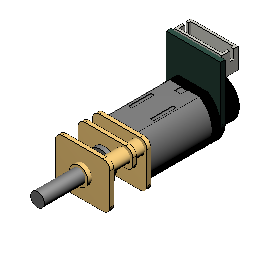
lf (Autodesk Fusion 360 archive; units mm, degrees)
design "N20-enc"
Autodesk Fusion 360 part; units mm, degrees
note: some values were not read from the file. Chosen so that the rebuilt part matches the saved one: a direction. Set by a fixed rule: which sketch regions a step uses.
sketch "Sketch1" plane through (0, 0, 0) normal (0, 1, 0) x (1, 0, 0)
  line L0 (-3.25, -5) -> (3.25, -5)
  arc A0 (3.25, -5) -> (3.25, 5) centre (0.0795, 0) ccw
  line L1 (3.25, 5) -> (-3.25, 5)
  arc A1 (-3.25, 5) -> (-3.25, -5) centre (-0.0795, 0) ccw
  line L2 (0, 0) -> (0, -6) construction
  line L3 (0, 0) -> (10, 0) construction
  dimension "d1" = 10
  dimension "d2" = 12
  dimension "d3" = 6.5
  constraint horizontal L0
  constraint horizontal L1
  constraint coincident L2.start L3.start
  constraint vertical L2
  constraint perpendicular L2 L3
  constraint symmetric L0 L1 L3
  constraint symmetric A0 A1 L2
  constraint equal L0 L1
  measures "d1" distance of L0 L1
  measures "d3" distance of L0.start L0.end
extrude "Extrude1" add sketch "Sketch1" along normal blind 13.5 makes body 1
extrude "Extrude2" add 1 faces at (1.0833, 13.5, -1.6667) along direction (0, 1, 0) blind 2 separate body on bodies 1 makes body 2
sketch "Sketch3" plane through (0, 0, 0) normal (0, -1, 0) x (1, 0, 0)
  arc A0 (-3.25, 5) -> (-3.25, -5) centre (-0.0795, 0) ccw
  line L0 (-3.25, -5) -> (3.25, -5)
  arc A1 (3.25, -5) -> (3.25, 5) centre (0.0795, 0) ccw
  line L1 (3.25, 5) -> (-3.25, 5)
  line L2 (-4.5, 5) -> (4.5, 5)
  line L3 (6, 3.5) -> (6, -3.5)
  line L4 (4.5, -5) -> (-4.5, -5)
  line L5 (-6, -3.5) -> (-6, 3.5)
  line L6 (0, 0) -> (0, 5) construction
  line L7 (0, 0) -> (6, 0) construction
  arc A2 (-4.5, 5) -> (-6, 3.5) centre (-4.5, 3.5) ccw
  arc A3 (6, 3.5) -> (4.5, 5) centre (4.5, 3.5) ccw
  arc A4 (4.5, -5) -> (6, -3.5) centre (4.5, -3.5) ccw
  arc A5 (-6, -3.5) -> (-4.5, -5) centre (-4.5, -3.5) ccw
  point P0 (-6, 5)
  point P1 (6, 5)
  point P2 (-6, -5)
  dimension "d8" = 12
  dimension "d9" = 10
  dimension "d10" = 1.5
  constraint horizontal L2
  constraint vertical L3
  constraint horizontal L4
  constraint vertical L5
  constraint vertical L6
  constraint coincident L6.start L7.start
  constraint perpendicular L3 L7
  constraint coincident L2 L6.end
  constraint coincident P0 L2
  constraint coincident P0 L5
  constraint tangent L2 A2
  constraint tangent L5 A2
  constraint coincident L3 L7.end
  constraint coincident P1 L2
  constraint coincident P1 L3
  constraint tangent L2 A3
  constraint tangent L3 A3
  constraint equal A2 A3
  constraint tangent L3 A4
  constraint tangent L4 A4
  constraint equal A2 A4
  constraint coincident P2 L4
  constraint coincident P2 L5
  constraint tangent L4 A5
  constraint tangent L5 A5
  constraint equal A2 A5
  constraint midpoint L2 L6.end
  constraint midpoint L3 L7.end
  measures "d8" distance of P0 P1
  measures "d9" distance of P0 P2
  measures "d10" radius of A2
extrude "Extrude3" add sketch "Sketch3" along normal blind 0.8 separate body makes body 3
sketch "Sketch4" plane through (0, 15.5, 0) normal (0, 1, 0) x (-1, 0, 0)
  arc A0 (3.25, -5) -> (3.25, 5) centre (0.0795, 0) ccw
  line L0 (3.25, 5) -> (-3.25, 5)
  arc A1 (-3.25, 5) -> (-3.25, -5) centre (-0.0795, 0) ccw
  line L1 (-6, 12) -> (-6, -1.5)
  line L2 (-6, 3.5) -> (-6, -3.5) construction
  line L3 (6, -3.5) -> (6, 3.5) construction
  line L4 (6, 12) -> (6, -1.5)
  line L5 (-6, 12) -> (6, 12)
  line L6 (-3.25, -5) -> (3.25, -5) construction
  line L7 (-4.25, -5) -> (4.25, -5)
  line L8 (-6, -1.5) -> (-4.25, -5)
  line L9 (4.25, -5) -> (6, -1.5)
  line L10 (0, 0) -> (0, 14.3086) construction
  circle A2 centre (0, 0) radius 1
  dimension "d13" = 17
  dimension "d14" = 8.5
  dimension "d15" = 13.5
  dimension "d18" = 2
  constraint vertical L1
  constraint collinear L1 L2
  constraint vertical L4
  constraint collinear L3 L4
  constraint horizontal L5
  constraint horizontal L7
  constraint collinear L6 L7
  constraint coincident L10.start A2.centre
  constraint vertical L10
  constraint symmetric L8 L9 L10
  measures "d13" distance of L5 L7
  measures "d14" distance of L7.start L7.end
  measures "d15" distance of L1.start L1.end
  measures "d18" diameter of A2
extrude "Extrude4" add sketch "Sketch4" along normal blind 1 separate body contours A0 L0 A1 L7 | A0 L0 A1 L1 L4 L5 makes body 4
sketch "Sketch5" plane through (0, 0, 0) normal (1, 0, 0) x (0, 1, 0)
  line L0 (24.2202, 0) -> (0, 0) construction
  line L1 (15, 0.5) -> (17.5, 0.5)
  line L2 (17.5, 0.5) -> (17.5, 4.6)
  line L3 (17.5, 4.6) -> (21, 4.6)
  line L4 (21, 4.6) -> (21, 2.6)
  line L5 (21, 2.6) -> (20.7, 1.5)
  line L6 (20.7, 1.5) -> (20.7, 0)
  line L7 (15, 0) -> (15, 0.5)
  line L8 (15, 0) -> (20.7, 0)
  dimension "d19" = 0.5
  dimension "d20" = 4.6
  dimension "d21" = 3.5
  dimension "d22" = 2
  dimension "d23" = 1.5
  dimension "d24" = 0.3
  dimension "d25" = 21
  dimension "d26" = 15
  constraint coincident L0.end origin
  constraint horizontal L0
  constraint parallel L0 L1
  constraint perpendicular L1 L2
  constraint perpendicular L2 L3
  constraint perpendicular L3 L4
  constraint coincident L0 L6.end
  constraint perpendicular L0 L6
  constraint coincident L0 L7.start
  constraint perpendicular L1 L7
  measures "d19" distance of L0 L1
  measures "d20" distance of L0 L3
  measures "d21" distance of L2.end L3.end
  measures "d22" distance of L3.end L4.end
  measures "d23" distance of L5.end L6.end
  measures "d24" distance of L4 L6
  measures "d25" distance of L0.end L4
  measures "d26" distance of L0.end L7
revolve "Revolve1" add sketch "Sketch5" angle 360 about axis through (0, 24.2202, 0) along (0, -1, 0) separate body makes body 5
sketch "Sketch6" plane through (0, 0, 0) normal (0, 1, 0) x (1, 0, 0)
  arc A0 (-4.5, 5) -> (-6, 3.5) centre (-4.5, 3.5) ccw
  line L0 (-6, 3.5) -> (-6, -3.5)
  arc A1 (-6, -3.5) -> (-4.5, -5) centre (-4.5, -3.5) ccw
  line L1 (-4.5, -5) -> (4.5, -5)
  arc A2 (4.5, -5) -> (6, -3.5) centre (4.5, -3.5) ccw
  line L2 (6, -3.5) -> (6, 3.5)
  arc A3 (6, 3.5) -> (4.5, 5) centre (4.5, 3.5) ccw
  line L3 (4.5, 5) -> (-4.5, 5)
  circle A4 centre (-4, 3) radius 1.5
  circle A5 centre (4, -3) radius 1.5
  arc A6 (-6, -3.5) -> (-4.5, -5) centre (-4.5, -3.5) ccw
  line L4 (-4.5, -5) -> (4.5, -5)
  arc A7 (4.5, -5) -> (6, -3.5) centre (4.5, -3.5) ccw
  line L5 (6, -3.5) -> (6, 3.5)
  arc A8 (6, 3.5) -> (4.5, 5) centre (4.5, 3.5) ccw
  line L6 (4.5, 5) -> (-4.5, 5)
  arc A9 (-4.5, 5) -> (-6, 3.5) centre (-4.5, 3.5) ccw
  line L7 (-6, 3.5) -> (-6, -3.5)
  dimension "d29" = 3
  dimension "d32" = 0.5
  dimension "d33" = 0.5
  dimension "d38" = 0.5
  dimension "d39" = 0.5
  constraint equal A4 A5
  measures "d29" diameter of A5
  measures "d32" distance of L2 A5
  measures "d33" distance of L0 A4
  measures "d38" distance of L3 A4
  measures "d39" distance of L1 A5
extrude "Extrude5" add sketch "Sketch6" against normal blind 8.5 from surface at -0.5 contours A4 | A5 bodies 3
sketch "Sketch8" plane through (0, -0.8, 0) normal (0, -1, 0) x (-1, 0, 0)
  line L0 (6, 3.5) -> (6, -3.5)
  arc A0 (6, 3.5) -> (4.5, 5) centre (4.5, 3.5) ccw
  arc A1 (-6, -3.5) -> (-4.5, -5) centre (-4.5, -3.5) ccw
  line L1 (4.5, -5) -> (-4.5, -5)
  arc A2 (4.5, -5) -> (6, -3.5) centre (4.5, -3.5) ccw
  line L2 (-1.0827, 4.0905) -> (-1.4214, 0.3651)
  line L3 (-2.2932, -0.5367) -> (-5.124, -0.8905)
  line L4 (4.5, 5) -> (-0.0868, 5)
  line L5 (-6, -3.5) -> (-6, -1.8828)
  arc A3 (-5.124, -0.8905) -> (-6, -1.8828) centre (-5, -1.8828) ccw
  arc A4 (-2.2932, -0.5367) -> (-1.4214, 0.3651) centre (-2.4172, 0.4556) ccw
  arc A5 (-0.0868, 5) -> (-1.0827, 4.0905) centre (-0.0868, 4) ccw
  point P0 (-1, 5)
  point P1 (-6, -1)
  dimension "d49" = 7
  dimension "d50" = 4
  dimension "d51" = 1
  constraint coincident A0.end L4.start
  constraint coincident A1.start L5.start
  constraint tangent A1 L5
  constraint coincident P1 L3
  constraint coincident P1 L5
  constraint tangent L3 A3
  constraint tangent L5 A3
  constraint tangent L2 A4
  constraint tangent L3 A4
  constraint equal A3 A4
  constraint coincident P0 L2
  constraint coincident P0 L4
  constraint tangent L2 A5
  constraint tangent L4 A5
  constraint equal A3 A5
  measures "d49" distance of L0 P0
  measures "d50" distance of L1 P1
  measures "d51" radius of A3
extrude "Extrude6" add sketch "Sketch8" along normal blind 0.8 from surface at 2.4 bodies 3
extrude "Extrude7" add sketch "Sketch3" against normal blind 0.8 from surface at 9 bodies 3
sketch "Sketch9" plane through (0, -9, 0) normal (0, -1, 0) x (1, 0, 0)
  line L0 (4.5, 5) -> (-4.5, 5)
  arc A0 (-4.5, 5) -> (-6, 3.5) centre (-4.5, 3.5) ccw
  line L1 (-6, 3.5) -> (-6, -3.5)
  arc A1 (-6, -3.5) -> (-4.5, -5) centre (-4.5, -3.5) ccw
  line L2 (-4.5, -5) -> (4.5, -5)
  arc A2 (4.5, -5) -> (6, -3.5) centre (4.5, -3.5) ccw
  line L3 (6, -3.5) -> (6, 3.5)
  arc A3 (6, 3.5) -> (4.5, 5) centre (4.5, 3.5) ccw
  circle A4 centre (0, 0) radius 2
  dimension "d55" = 4
  constraint coincident A4.centre origin
  measures "d55" diameter of A4
extrude "Extrude8" add sketch "Sketch9" along normal blind 0.9 contours A4 bodies 3
sketch "Sketch10" plane through (0, 0, 0) normal (1, 0, 0) x (0, 1, 0)
  line L0 (-19, 1.5) -> (-8.2, 1.5)
  line L1 (-19, 0) -> (-19, 1.5)
  line L2 (-8.2, 1.5) -> (-8.2, 2)
  line L3 (-8.2, 2) -> (-5.2, 2)
  line L4 (0, 0) -> (-19, 0) construction
  line L5 (-4.2, 2.75) -> (-5.2, 2.75)
  line L6 (-4.2, 0.5) -> (-3.2, 0.5)
  line L7 (-3.2, 0.5) -> (-3.2, 0)
  line L8 (-5.2, 2.75) -> (-5.2, 2)
  line L9 (-3.2, -3.5) -> (-3.2, 3.5) construction
  line L10 (-4, 3.5) -> (-4, -3.5) construction
  line L11 (-8.2, -3.5) -> (-8.2, 3.5) construction
  line L12 (-9, -3.5) -> (-9, 3.5) construction
  line L13 (-4.2, 0.5) -> (-4.2, 2.75)
  line L14 (-19, 0) -> (-3.2, 0)
  dimension "d62" = 3
  dimension "d64" = 10
  dimension "d65" = 1.5
  dimension "d66" = 2
  dimension "d67" = 2.75
  dimension "d68" = 0.5
  dimension "d69" = 0.2
  constraint horizontal L0
  constraint vertical L1
  constraint perpendicular L0 L2
  constraint coincident L4.start origin
  constraint horizontal L5
  constraint vertical L8
  constraint horizontal L6
  constraint vertical L7
  constraint collinear L7 L9
  constraint collinear L2 L11
  measures "d62" distance of L2 L8
  measures "d64" distance of L1 L12
  measures "d65" distance of L0 L4
  measures "d66" distance of L3 L14
  measures "d67" distance of L4 L5
  measures "d68" distance of L6 L14
  measures "d69" distance of L10 L13
revolve "Revolve2" add sketch "Sketch10" angle 360 about axis through (0, 0, 0) along (0, -1, 0) separate body makes body 6
sketch "Sketch11" plane through (0, 16.5, 0) normal (0, 1, 0) x (-1, 0, 0)
  circle A0 centre (0, 0) radius 1
  line L0 (-6, 12) -> (-6, 0)
  arc A1 (-6, 0) -> (-3.25, -5) centre (-0.0795, 0) ccw
  line L1 (-3.25, -5) -> (3.25, -5)
  arc A2 (3.25, -5) -> (6, 0) centre (0.0795, 0) ccw
  line L2 (6, 0) -> (6, 12)
  line L3 (6, 12) -> (-6, 12)
  line L4 (-5.25, 12.4) -> (5.25, 12.4)
  line L5 (5.25, 12.4) -> (5.25, 7.9)
  line L6 (5.25, 7.9) -> (-5.25, 7.9)
  line L7 (-5.25, 7.9) -> (-5.25, 12.4)
  line L8 (0, 0) -> (0, 18.1441) construction
  dimension "d71" = 4.5
  dimension "d72" = 10.5
  dimension "d73" = 0.4
  constraint horizontal L4
  constraint vertical L5
  constraint horizontal L6
  constraint vertical L7
  constraint coincident A0.centre L8.start
  constraint vertical L8
  constraint symmetric L5 L7 L8
  measures "d71" distance of L4.end L5.end
  measures "d72" distance of L4.start L4.end
  measures "d73" distance of L3 L4
extrude "Extrude9" add sketch "Sketch11" along normal blind 3.6 separate body contours L3 L4 L5 L7 | L3 L5 L6 L7 makes body 7
sketch "Sketch12" plane through (0, 0, 12.4) normal (0, 0, 1) x (-1, 0, 0)
  line L0 (5.25, -16.5) -> (-5.25, -16.5)
  line L1 (-5.25, -16.5) -> (-5.25, -20.1)
  line L2 (-5.25, -20.1) -> (5.25, -20.1)
  line L3 (5.25, -20.1) -> (5.25, -16.5)
  line L4 (4.75, -19.6) -> (4.75, -17)
  line L5 (4.75, -17) -> (-4.75, -17)
  line L6 (-4.75, -17) -> (-4.75, -19.6)
  line L7 (-4.75, -19.6) -> (4.75, -19.6)
  dimension "d76" = -0.5
extrude "Extrude10" cut sketch "Sketch12" against normal blind 3.3 contours L4 L5 L6 L7 bodies 7
sketch "Sketch13" plane through (5.25, 0, 0) normal (1, 0, 0) x (0, 1, 0)
  line L0 (16.5, 7.9) -> (20.1, 7.9)
  line L1 (20.1, 7.9) -> (20.1, 12.4)
  line L2 (20.1, 12.4) -> (16.5, 12.4)
  line L3 (16.5, 12.4) -> (16.5, 7.9)
  line L4 (18.25, 12.4) -> (19.1, 12.4)
  line L5 (19.1, 12.4) -> (19.1, 10.4)
  line L6 (19.1, 10.4) -> (18.25, 10.4)
  line L7 (18.25, 10.4) -> (18.25, 12.4)
  dimension "d79" = 1
  dimension "d80" = 0.85
  dimension "d81" = 2.5
  constraint horizontal L4
  constraint vertical L5
  constraint horizontal L6
  constraint vertical L7
  constraint coincident L2 L4.start
  measures "d79" distance of L1 L5
  measures "d80" distance of L5.end L6.end
  measures "d81" distance of L0 L6
extrude "Extrude11" cut sketch "Sketch13" against normal through all contours L2 L4 L5 L6 L7 bodies 7
sketch "Sketch14" plane through (0, 0, 5) normal (0, 0, 1) x (-1, 0, 0)
  line L0 (3.25, 0) -> (-3.25, 0)
  line L1 (-3.25, 0) -> (-3.25, -13.5)
  line L2 (-3.25, -13.5) -> (3.25, -13.5)
  line L3 (3.25, -13.5) -> (3.25, 0)
  line L4 (2.8, -8.9) -> (2.05, -8.9)
  line L5 (2.05, -8.9) -> (2.05, -3.9)
  line L6 (2.05, -3.9) -> (2.8, -3.9)
  line L7 (2.8, -3.9) -> (2.8, -8.9)
  line L8 (-2.05, -8.9) -> (-2.8, -8.9)
  line L9 (-2.8, -8.9) -> (-2.8, -3.9)
  line L10 (-2.8, -3.9) -> (-2.05, -3.9)
  line L11 (-2.05, -3.9) -> (-2.05, -8.9)
  line L12 (0.7, -13.5) -> (-0.7, -13.5)
  line L13 (-0.7, -13.5) -> (-0.7, -12)
  line L14 (-0.7, -12) -> (0.7, -12)
  line L15 (0.7, -12) -> (0.7, -13.5)
  line L16 (0, 0) -> (0, -22.5) construction
  dimension "d83" = 0.75
  dimension "d84" = 4.1
  dimension "d85" = 3.9
  dimension "d86" = 5
  dimension "d87" = 1.5
  dimension "d88" = 1.4
  constraint horizontal L4
  constraint vertical L5
  constraint horizontal L6
  constraint vertical L7
  constraint horizontal L8
  constraint vertical L9
  constraint horizontal L10
  constraint vertical L11
  constraint horizontal L12
  constraint vertical L13
  constraint horizontal L14
  constraint vertical L15
  constraint coincident L2 L12.start
  constraint coincident L16.start origin
  constraint perpendicular L0 L16
  constraint collinear L4 L8
  constraint collinear L6 L10
  measures "d83" distance of L5 L7
  measures "d84" distance of L5 L11
  measures "d85" distance of L0 L6
  measures "d86" distance of L4.end L5.end
  measures "d87" distance of L12.end L13.end
  measures "d88" distance of L13.end L14.end
extrude "Extrude12" cut sketch "Sketch14" against normal blind 0.2 contours L2 L12 L13 L14 L15 | L4 L5 L6 L7 | L8 L9 L10 L11 bodies 1
extrude "Extrude13" cut sketch "Sketch14" along normal blind 0.2 from surface at -10 contours L4 L5 L6 L7 | L8 L9 L10 L11 bodies 1
equation "d20 = ( 9.2 / 2 ) * 1 mm"

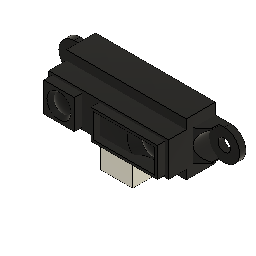
design "GY-521"
Autodesk Fusion 360 part; units mm, degrees
sketch "Sketch3" plane through (0, 0, 0) normal (1, 0, 0) x (0, 1, 0)
  line L0 (0, 6.5) -> (0, -6.5)
  line L1 (0, -6.5) -> (-7.15, -6.5)
  line L2 (-7.15, -6.5) -> (-7.15, -4.2)
  line L3 (-7.15, -4.2) -> (-11.5, -4.2)
  line L4 (-11.5, -4.2) -> (-11.5, -3.625)
  line L5 (-11.5, -3.625) -> (-13.5, -3.625)
  line L6 (-13.5, -3.625) -> (-13.5, 3.625)
  line L7 (-13.5, 3.625) -> (-11.5, 3.625)
  line L8 (-11.5, 3.625) -> (-11.5, 4.2)
  line L9 (-11.5, 4.2) -> (-7.15, 4.2)
  line L10 (-7.15, 4.2) -> (-7.15, 6.5)
  line L11 (-7.15, 6.5) -> (0, 6.5)
  line L12 (0, 0) -> (-13.5, 0) construction
  dimension "d5" = 13
  dimension "d6" = 8.4
  dimension "d7" = 7.25
  dimension "d8" = 7.15
  dimension "d9" = 11.5
  dimension "d10" = 13.5
  constraint vertical L0
  constraint perpendicular L0 L1
  constraint perpendicular L1 L2
  constraint perpendicular L2 L3
  constraint perpendicular L1 L4
  constraint perpendicular L4 L5
  constraint perpendicular L5 L6
  constraint perpendicular L6 L7
  constraint perpendicular L5 L8
  constraint perpendicular L6 L9
  constraint perpendicular L9 L10
  constraint perpendicular L0 L11
  constraint midpoint L12.start L0
  constraint coincident L12.start origin
  constraint midpoint L6 L12.end
  constraint horizontal L12
  constraint collinear L2 L10
  constraint collinear L4 L8
  constraint symmetric L3 L9 L12
  measures "d5" distance of L0.start L0.end
  measures "d6" distance of L3 L9
  measures "d7" distance of L5 L7
  measures "d8" distance of L0 L10
  measures "d9" distance of L0 L8
  measures "d10" distance of L0 L6
extrude "Extrude2" add sketch "Sketch3" along normal mid plane 29.5 makes body 1
sketch "Sketch4" plane through (0, 0, 6.5) normal (0, 0, 1) x (-1, 0, 0)
  line L0 (14.75, 7.15) -> (-14.75, 7.15)
  line L1 (-14.75, 7.15) -> (-14.75, 0)
  line L2 (-14.75, 0) -> (14.75, 0)
  line L3 (14.75, 0) -> (14.75, 7.15)
  line L4 (14.75, 11.5) -> (-14.75, 11.5)
  line L5 (14.75, 13.5) -> (13.97, 13.5)
  line L6 (13.97, 13.5) -> (13.97, 11.5)
  line L7 (13.97, 11.5) -> (14.75, 11.5)
  line L8 (14.75, 11.5) -> (14.75, 13.5)
  line L9 (-14.75, 13.5) -> (-13.97, 13.5)
  line L10 (-13.97, 13.5) -> (-13.97, 11.5)
  line L11 (-13.97, 11.5) -> (-14.75, 11.5)
  line L12 (-14.75, 11.5) -> (-14.75, 13.5)
  line L13 (6.47, 11.5) -> (2.33, 11.5)
  line L14 (2.33, 11.5) -> (2.33, 13.5)
  line L15 (2.33, 13.5) -> (6.47, 13.5)
  line L16 (6.47, 13.5) -> (6.47, 11.5)
  point P0 (14.75, 13.5)
  point P1 (-14.75, 13.5)
  dimension "d13" = 0.78
  dimension "d14" = 7.5
  dimension "d15" = 16.3
  constraint horizontal L5
  constraint vertical L6
  constraint horizontal L7
  constraint vertical L8
  constraint coincident P0 L5.start
  constraint horizontal L9
  constraint vertical L10
  constraint horizontal L11
  constraint vertical L12
  constraint coincident L4 L10.end
  constraint coincident P1 L9.start
  constraint horizontal L13
  constraint vertical L14
  constraint horizontal L15
  constraint vertical L16
  constraint coincident L4 L13.start
  constraint collinear L9 L15
  constraint collinear L4 L7
  constraint equal L5 L9
  measures "d13" distance of P0 L5.end
  measures "d14" distance of L6 L16
  measures "d15" distance of L10 L14
extrude "Extrude3" cut sketch "Sketch4" against normal through all contours L4 L5 L6 L7 L8 | L4 L13 L14 L15 L16 | L4 L9 L10 L11 L12 bodies 1
sketch "Sketch5" plane through (0, 0, 0) normal (0, 1, 0) x (-1, 0, 0)
  line L0 (14.75, 6.5) -> (-14.75, 6.5)
  line L1 (-14.75, 6.5) -> (-14.75, -6.5)
  line L2 (-14.75, -6.5) -> (14.75, -6.5)
  line L3 (14.75, -6.5) -> (14.75, 6.5)
  line L4 (14, -5.75) -> (14, 5.75)
  line L5 (14, 5.75) -> (-14, 5.75)
  line L6 (-14, 5.75) -> (-14, -5.75)
  line L7 (5.5, -5.75) -> (5.5, -6.5)
  line L8 (5.5, -6.5) -> (-5.5, -6.5)
  line L9 (-5.5, -6.5) -> (-5.5, -5.75)
  line L10 (-14, -5.75) -> (-5.5, -5.75)
  line L11 (5.5, -5.75) -> (14, -5.75)
  line L12 (0, -6.5) -> (0, 5.75) construction
  dimension "d18" = 0.75
  dimension "d20" = 0.75
  dimension "d21" = 0.75
  dimension "d22" = 11
  constraint vertical L7
  constraint horizontal L8
  constraint vertical L9
  constraint parallel L2 L10
  constraint parallel L3 L4
  constraint parallel L0 L5
  constraint parallel L1 L6
  constraint collinear L10 L11
  constraint midpoint L8 L12.start
  constraint midpoint L5 L12.end
  constraint coincident origin L12
  constraint vertical L12
  constraint collinear L2 L8
  measures "d18" distance of L1 L6
  measures "d20" distance of L0 L5
  measures "d21" distance of L2 L10
  measures "d22" distance of L7.end L8.end
extrude "Extrude4" cut sketch "Sketch5" against normal blind 4.5 contours L2 L4 L5 L6 L7 L8 L9 L10 L11 bodies 1
sketch "Sketch6" plane through (0, 0, 0) normal (0, 0, 1) x (1, 0, 0)
  arc A0 (-12.47, -12.5) -> (-10.22, -13) centre (-10.22, -7.6875) ccw
  line L0 (-13.97, -13.5) -> (-6.47, -13.5)
  line L1 (-12.47, -12.5) -> (-13.22, -13.5)
  line L2 (-10.22, -13) -> (-10.22, -13.5)
  line L3 (-13.22, -13.5) -> (-10.22, -13.5)
  line L4 (-10.22, -13) -> (-8.3686, -13) construction
  dimension "d25" = 0.5
  dimension "d26" = 3
  dimension "d27" = 2.25
  dimension "d28" = 1
  constraint coincident L0 L1.end
  constraint midpoint L0 L2.end
  constraint vertical L2
  constraint horizontal L4
  constraint tangent A0 L4
  measures "d25" distance of A0 L0
  measures "d26" distance of L1.end L2
  measures "d27" distance of A0.start L2
  measures "d28" distance of A0.start L3
revolve "Revolve1" cut sketch "Sketch6" angle 360 about axis through (-10.22, -13, 0) along (0, -1, 0) bodies 1
sketch "Sketch7" plane through (0, -13.5, 0) normal (0, -1, 0) x (1, 0, 0)
  line L0 (-2.33, 3.625) -> (-2.33, -3.625)
  line L1 (-2.33, -3.625) -> (13.97, -3.625)
  line L2 (13.97, -3.625) -> (13.97, 3.625)
  line L3 (13.97, 3.625) -> (-2.33, 3.625)
  line L4 (-1.73, 3.025) -> (13.37, 3.025)
  line L5 (13.37, 3.025) -> (13.37, -3.025)
  line L6 (13.37, -3.025) -> (-1.73, -3.025)
  line L7 (-1.73, -3.025) -> (-1.73, 3.025)
  dimension "d30" = 0.6
  dimension "d31" = 0.6
  dimension "d32" = 0.6
  dimension "d33" = 0.6
  constraint horizontal L4
  constraint vertical L5
  constraint horizontal L6
  constraint vertical L7
  measures "d30" distance of L0 L7
  measures "d31" distance of L3 L4
  measures "d32" distance of L2 L5
  measures "d33" distance of L1 L6
extrude "Extrude5" cut sketch "Sketch7" against normal blind 1.7 contours L4 L5 L6 L7 bodies 1
extrude "Extrude6" add 1 faces at (8.3367, -11.8, -1.0083) along direction (0, 1, 0) blind 2 separate body on bodies 1 makes body 2
sketch "Sketch8" plane through (0, 0, 0) normal (0, 0, 1) x (1, 0, 0)
  line L0 (9.47, -13.5) -> (9.47, -10.9)
  line L1 (13.97, -11.5) -> (13.97, -13.5)
  line L2 (4.97, -11.8) -> (6.72, -10.05)
  line L3 (-1.73, -11.8) -> (13.37, -11.8) construction
  line L4 (13.37, -11.8) -> (-1.73, -11.8)
  line L5 (9.47, -10.9) -> (16.1613, -10.9) construction
  line L6 (-2.33, -13.5) -> (13.97, -13.5)
  arc A0 (6.72, -10.05) -> (9.47, -10.9) centre (9.47, -6.0265) ccw
  dimension "d38" = 4.5
  dimension "d39" = 4.5
  dimension "d40" = 2.6
  dimension "d41" = 2.75
  dimension "d42" = 45
  constraint vertical L0
  constraint coincident L2.start L4
  constraint perpendicular L0 L5
  constraint tangent L5 A0
  measures "d38" distance of L0 L1
  measures "d39" distance of L0 L2.start
  measures "d40" distance of L5 L6
  measures "d41" distance of L0 L2.end
  measures "d42" angle of L2 L4
revolve "Revolve2" cut sketch "Sketch8" angle 360 about axis through (9.47, -13.5, 0) along (0, 1, 0) keep common part bodies 2
combine "Combine1" operation cut target body 1 tool bodies 2
sketch "Sketch9" plane through (0, 0, 0) normal (0, 0, 1) x (1, 0, 0)
  line L0 (-14.75, 0) -> (-14.75, -7.15) construction
  line L1 (14.75, -7.15) -> (14.75, 0)
  line L2 (-14.75, 0) -> (-22.25, 0)
  line L3 (-22.25, 0) -> (-22.25, -1.5)
  line L4 (-22.25, -1.5) -> (-17.15, -1.5)
  line L5 (-17.15, -1.5) -> (-17.15, -3.2)
  line L6 (-17.15, -3.2) -> (-14.75, -5.5)
  line L7 (-14.75, 0) -> (-14.75, -5.5)
  dimension "d44" = 1.5
  dimension "d45" = 22.25
  dimension "d46" = 17.15
  dimension "d47" = 5.5
  dimension "d48" = 3.2
  constraint coincident L0.start L2.start
  constraint perpendicular L0 L2
  constraint perpendicular L2 L3
  constraint perpendicular L3 L4
  constraint perpendicular L4 L5
  constraint coincident L0 L6.end
  measures "d44" distance of L2.end L3.end
  measures "d45" distance of origin L3
  measures "d46" distance of origin L5
  measures "d47" distance of L0.start L6.end
  measures "d48" distance of L2 L5.end
extrude "Extrude7" add sketch "Sketch9" along normal mid plane 7.5 bodies 1
sketch "Sketch10" plane through (0, -1.5, 0) normal (0, -1, 0) x (1, 0, 0)
  line L0 (-17.15, -3.75) -> (-17.15, 3.75)
  line L1 (-17.15, 3.75) -> (-22.25, 3.75)
  line L2 (-22.25, 3.75) -> (-22.25, -3.75)
  line L3 (-22.25, -3.75) -> (-17.15, -3.75)
  circle A0 centre (-18.5, 0) radius 3.75
  dimension "d51" = 18.5
  constraint horizontal origin A0.centre
  constraint tangent L2 A0
  constraint tangent L1 A0
  measures "d51" distance of origin A0.centre
extrude "Extrude8" cut sketch "Sketch10" along normal through all contours L0 A0 | L0 A0 bodies 1
sketch "Sketch11" plane through (0, -1.5, 0) normal (0, -1, 0) x (1, 0, 0)
  line L0 (-17.15, -3.75) -> (-17.15, -3.4986)
  arc A0 (-17.15, -3.4986) -> (-17.15, 3.4986) centre (-18.5, 0) ccw
  line L1 (-17.15, 3.4986) -> (-17.15, 3.75)
  line L2 (-17.15, 3.75) -> (-22.25, 3.75)
  line L3 (-22.25, 3.75) -> (-22.25, -3.75)
  line L4 (-22.25, -3.75) -> (-17.15, -3.75)
  arc A1 (-18.5, 3.75) -> (-18.5, -3.75) centre (-18.5, 0) ccw
  line L5 (-18.5, 3.75) -> (-23.25, 3.75)
  line L6 (-23.25, 3.75) -> (-23.25, -3.75)
  line L7 (-18.5, -3.75) -> (-23.25, -3.75)
  circle A2 centre (-18.5, 0) radius 1.55
  dimension "d53" = 1
  dimension "d54" = 3.1
  constraint equal A0 A1
  constraint concentric A0 A1
  constraint coincident L4 A1.end
  constraint coincident L2 A1.start
  constraint tangent A1 L5
  constraint perpendicular L3 L5
  constraint perpendicular L5 L6
  constraint horizontal L7
  constraint concentric A0 A2
  measures "d53" distance of A1 L6
  measures "d54" diameter of A2
extrude "Extrude9" cut sketch "Sketch11" against normal through all contours L3 L4 A1 L7 | L2 L3 A1 L5 | A2 bodies 1
mirror "Mirror1" about plane through (0, 0, 0) normal (1, 0, 0) of "Extrude7", "Extrude8", "Extrude9"
sketch "Sketch13" plane through (0, -7.15, 0) normal (0, -1, 0) x (1, 0, 0)
  line L0 (-14.75, -6.5) -> (14.75, -6.5)
  line L1 (14.75, -6.5) -> (14.75, -4.2)
  line L2 (14.75, -4.2) -> (-14.75, -4.2)
  line L3 (-14.75, -4.2) -> (-14.75, -6.5)
  line L4 (-5.5, -4.2) -> (5.5, -4.2)
  line L5 (5.5, -4.2) -> (5.5, -6.5)
  line L6 (5.5, -6.5) -> (-5.5, -6.5)
  line L7 (-5.5, -6.5) -> (-5.5, -4.2)
  point P0 (-5.5, -6.5)
  point P1 (5.5, -6.5)
  constraint horizontal L4
  constraint vertical L5
  constraint horizontal L6
  constraint vertical L7
  constraint coincident L0 P1
  constraint collinear L2 L4
  constraint coincident P1 L5.end
  constraint coincident P0 L6.end
extrude "Extrude10" cut sketch "Sketch13" against normal through all contours L0 L2 L4 L5 L6 L7 bodies 1
sketch "Sketch14" plane through (0, -4.5, 0) normal (0, 1, 0) x (-1, 0, 0)
  line L0 (5.5, -4.2) -> (5.5, -5.75)
  line L1 (5.5, -5.75) -> (14, -5.75)
  line L2 (14, -5.75) -> (14, 5.75)
  line L3 (14, 5.75) -> (-14, 5.75)
  line L4 (-14, 5.75) -> (-14, -5.75)
  line L5 (-14, -5.75) -> (-5.5, -5.75)
  line L6 (-5.5, -5.75) -> (-5.5, -4.2)
  line L7 (-5.5, -4.2) -> (5.5, -4.2)
  line L8 (-13.8, 5.55) -> (13.8, 5.55)
  line L9 (13.8, 5.55) -> (13.8, -5.55)
  line L10 (-13.8, -5.55) -> (-13.8, 5.55)
  line L11 (5.05, -5.55) -> (5.05, -12.5)
  line L12 (5.05, -12.5) -> (-5.05, -12.5)
  line L13 (-5.05, -12.5) -> (-5.05, -5.55)
  line L14 (13.8, -5.55) -> (5.05, -5.55)
  line L15 (-5.05, -5.55) -> (-13.8, -5.55)
  line L16 (0, 5.55) -> (0, -12.5) construction
  line L17 (14.75, 6.5) -> (-14.75, 6.5)
  dimension "d59" = 0.2
  dimension "d60" = 0.2
  dimension "d61" = 0.2
  dimension "d62" = 19
  dimension "d63" = 10.1
  constraint horizontal L8
  constraint vertical L9
  constraint horizontal L14
  constraint vertical L10
  constraint vertical L11
  constraint horizontal L12
  constraint vertical L13
  constraint coincident L13.end L14
  constraint collinear L14 L15
  constraint midpoint L8 L16.start
  constraint midpoint L12 L16.end
  constraint coincident origin L16
  constraint vertical L16
  measures "d59" distance of L4 L10
  measures "d60" distance of L3 L8
  measures "d61" distance of L5 L15
  measures "d62" distance of L12 L17
  measures "d63" distance of L11.end L12.end
extrude "Extrude11" add sketch "Sketch14" along normal up to surface (1.2 mm away) separate body contours L0 L6 L7 L8 L9 L10 L14 L15 | L0 L6 L7 L11 L12 L13 L14 L15 makes body 3
sketch "Sketch15" plane through (0, -4.5, 0) normal (0, -1, 0) x (1, 0, 0)
  line L0 (5.05, -12.5) -> (5.05, -5.55)
  line L1 (5.05, -5.55) -> (13.8, -5.55)
  line L2 (13.8, -5.55) -> (13.8, 5.55)
  line L3 (13.8, 5.55) -> (-13.8, 5.55)
  line L4 (-13.8, 5.55) -> (-13.8, -5.55)
  line L5 (-13.8, -5.55) -> (-5.05, -5.55)
  line L6 (-5.05, -5.55) -> (-5.05, -12.5)
  line L7 (-5.05, -12.5) -> (5.05, -12.5)
  line L8 (-2.9, -6.5) -> (2.9, -6.5)
  line L9 (3.9, -6.5) -> (3.9, -12.5)
  line L10 (3.9, -12.5) -> (-3.9, -12.5)
  line L11 (-3.9, -12.5) -> (-3.9, -6.5)
  line L12 (0, 0) -> (0, -6.5) construction
  line L13 (-3.9, -4.9) -> (-2.9, -4.9)
  line L14 (-2.9, -4.9) -> (-2.9, -6.5)
  line L15 (-3.9, -6.5) -> (-3.9, -4.9)
  line L16 (3.9, -6.5) -> (3.9, -4.9)
  line L17 (3.9, -4.9) -> (2.9, -4.9)
  line L18 (2.9, -4.9) -> (2.9, -6.5)
  dimension "d67" = 7.8
  dimension "d68" = 6
  dimension "d69" = 7.6
  dimension "d70" = 1
  constraint horizontal L8
  constraint vertical L9
  constraint horizontal L10
  constraint vertical L11
  constraint coincident L7 L9.end
  constraint coincident L12.start origin
  constraint vertical L12
  constraint horizontal L13
  constraint vertical L14
  constraint vertical L15
  constraint collinear L11 L15
  constraint perpendicular L8 L16
  constraint perpendicular L9 L17
  constraint perpendicular L8 L18
  constraint collinear L13 L17
  constraint equal L13 L17
  constraint coincident L8 L12.end
  constraint midpoint L8 L12.end
  measures "d67" distance of L9.end L10.end
  measures "d68" distance of L8 L10
  measures "d69" distance of L10 L13
  measures "d70" distance of L13.start L13.end
extrude "Extrude12" add sketch "Sketch15" along normal blind 5 separate body contours L7 L8 L9 L10 L11 L13 L14 L15 L16 L17 L18 makes body 4
